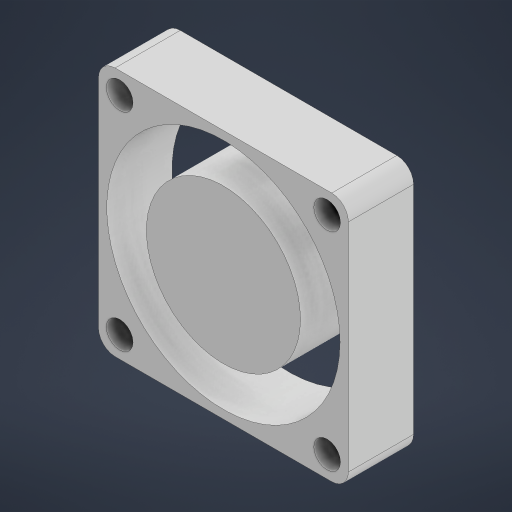
# Autodesk Inventor part: Fan
Saved by Autodesk Inventor 2024 (Build 280153000, 153)
## iProperties
Created: 2025-09-25
Part Number: Fan
Material: Generic
Document SubType Name: Modeling
Designer: kevin
Density: 1 g/cm^3
Appearance: Default
Author: kevin
Autodesk Inventor part; units mm, degrees
ref_plane "YZ Plane" through (0, 0, 0) normal (1, 0, 0) x (0, 1, 0)
ref_plane "XZ Plane" through (0, 0, 0) normal (0, 1, 0) x (-1, 0, 0)
ref_plane "XY Plane" through (0, 0, 0) normal (0, 0, 1) x (1, 0, 0)
sketch "Sketch1" plane through (0, 0, 0) normal (0, 0, 1) x (1, 0, 0)
  line L0 (-15, -15) -> (15, -15)
  line L1 (15, -15) -> (15, 15)
  line L2 (15, 15) -> (-15, 15)
  line L3 (-15, 15) -> (-15, -15)
  line L4 (-15, -15) -> (15, 15) construction
  line L5 (15, -15) -> (-15, 15) construction
  circle A0 centre (-12.45, 12.45) radius 1.6
  line L6 (0, 15) -> (0, 0) construction
  line L7 (0, 0) -> (-15, 0) construction
  circle A1 centre (12.45, 12.45) radius 1.6
  circle A2 centre (-12.45, -12.45) radius 1.6
  circle A3 centre (12.45, -12.45) radius 1.6
  circle A4 centre (0, 0) radius 14
  circle A5 centre (0, 0) radius 9.25
  dimension "d0" = 30
  dimension "d1" = 30
  dimension "d2" = 3.2
  dimension "d3" = 2.55
  dimension "d4" = 2.55
  dimension "d5" = 28
  dimension "d6" = 18.5
  constraints: 16 end point, 6 centre point, 4 midpoint, 3 symmetric about line, 2 coincident, 2 parallel, 1 horizontal, 1 perpendicular, 1 vertical, 3 other
  measures "d0" distance of L2.end L1.end
  measures "d1" distance of L1.end L0.end
  measures "d2" diameter of A0
  measures "d3" distance from line of L2 A0.centre
  measures "d4" distance from line of L3 A0.centre
  measures "d5" diameter of A4
  measures "d6" diameter of A5
extrude "Extrusion1" add sketch "Sketch1" along normal blind 7.82
fillet "Fillet1" radius 2 4 edges at (15, 15, 3.91) (-15, 15, 3.91) (-15, -15, 3.91) (15, -15, 3.91)
equation "\"d4\" = d3"
body "Solid1"
